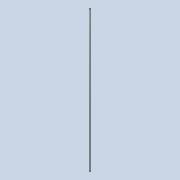
# Autodesk Inventor part: TUBO REDONDO INOX 304 OD 1/2" (Ø12,7 mm x 2 mm) - 1500 mm
Saved by Autodesk Inventor 2020 (Build 240168000, 168)
## iProperties
Manager: MARCOS SILVA
RuleStatus: InUse
Created: 2025-12-11
Part Number: TUBO REDONDO INOX 304 OD 1/2" (Ø12,7 mm x 2 mm) - 1500 mm
Cost Center: Nº DO ITEM
Material: Aço inoxidável, austenítico
Catalog Web Link: www.doma.ind.br
Vendor: DOMA TECNOLOGIA EM EQUIPAMENTOS INDUSTRIAIS
Document SubType Name: Modeling
Designer: JOAHAN
Stock Number: TUBO REDONDO
Mass: 806.761 g
Surface Area: 1009.8 cm^2
Volume: 100.845 cm^3
Density: 8 g/cm^3
Appearance: Semipolido
Ø: 12,700 mm
Thickness: 2,000 mm
COMPRIMENTO: 1500,000 mm
Subject: Standard (mm)
Author: JOAHAN
Autodesk Inventor part; units mm, degrees
ref_plane "YZ Plane" through (0, 0, 0) normal (1, 0, 0) x (0, 1, 0)
ref_plane "XZ Plane" through (0, 0, 0) normal (0, 1, 0) x (-1, 0, 0)
ref_plane "XY Plane" through (0, 0, 0) normal (0, 0, 1) x (1, 0, 0)
sketch "Esboço1" plane through (0, 0, 0) normal (0, 1, 0) x (-1, 0, 0)
  circle A0 centre (0, 0) radius 6.35
  circle A1 centre (0, 0) radius 4.35
  dimension "d0" = 12.7
  dimension "d1" = 2
  constraints: 2 centre point, 1 coincident
  measures "d0" diameter of A0
  measures "d1" radial gap between concentric circles of A0 A1
extrude "Extrusão1" add sketch "Esboço1" along normal mid plane 1500
equation "\"Ø\" = d0"
equation "\"Thickness\" = d1"
equation "\"COMPRIMENTO\" = d2"
equation "\"d2\" = 1500"
